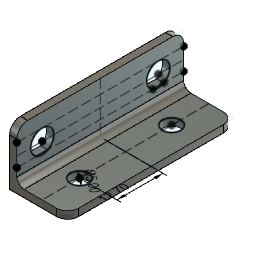
WideBaseAntennaMount (Autodesk Fusion 360 design; units mm, degrees)
Autodesk Fusion 360 part; units mm, degrees
note: some values were not read from the file. Set by a fixed rule: which sketch regions a step uses.
sketch "Sketch1" plane through (0, 0, 0) normal (0, 0, 1) x (1, 0, 0)
  line L0 (0, 0) -> (16, 0)
  line L1 (16, 0) -> (16, 2)
  line L2 (16, 2) -> (2, 2)
  line L3 (2, 2) -> (2, 16)
  line L4 (2, 16) -> (0, 16)
  line L5 (0, 16) -> (0, 0)
  dimension "d1" = 16
  dimension "d2" = 16
  dimension "d3" = 2
  dimension "d4" = 2
  constraint coincident L0.start L5.end
  constraint horizontal L0
  constraint perpendicular L0 L1
  constraint perpendicular L1 L2
  constraint perpendicular L2 L3
  constraint perpendicular L3 L4
  constraint perpendicular L0 L5
  measures "d1" distance of L4.end L0.start
  measures "d2" distance of L0.start L0.end
  measures "d3" distance of L0.end L1.end
  measures "d4" distance of L3.end L4.end
extrude "Extrude1" add sketch "Sketch1" against normal blind 46
sketch "Sketch2" plane through (0, 2, 0) normal (0, 1, 0) x (-1, 0, 0)
  line L0 (-2, 0) -> (-16, 0)
  line L1 (-16, 0) -> (-16, -46)
  line L2 (-16, -46) -> (-2, -46)
  line L3 (-2, -46) -> (-2, 0)
  line L4 (-9, -46) -> (-9, 0) construction
  line L5 (-16, -23) -> (-2, -23) construction
  circle A0 centre (-9, -10.3) radius 2.5
  circle A1 centre (-9, -35.7) radius 2.5
  dimension "d7" = 5
  dimension "d19" = 12.7
  constraint midpoint L2 L4.start
  constraint midpoint L0 L4.end
  constraint midpoint L1 L5.start
  constraint midpoint L3 L5.end
  constraint coincident L4 A0.centre
  constraint symmetric L5 A0 A1
  measures "d7" diameter of A0
  measures "d19" distance of L5 A0.centre
extrude "Extrude2" cut sketch "Sketch2" against normal blind 2 contours A0 | A1
sketch "Sketch3" plane through (2, 0, 0) normal (1, 0, 0) x (0, 0, -1)
  line L0 (0, 16) -> (0, 2)
  line L1 (0, 2) -> (46, 2)
  line L2 (46, 2) -> (46, 16)
  line L3 (46, 16) -> (0, 16)
  line L4 (23, 16) -> (23, 2) construction
  line L5 (0, 9) -> (46, 9) construction
  circle A0 centre (7, 9) radius 3.2
  line L6 (0, 12.2) -> (46, 12.2) construction
  line L7 (0, 6.2) -> (46, 6.2) construction
  line L8 (5.4508, 6.2) -> (8.5492, 6.2)
  circle A1 centre (39, 9) radius 3.2
  line L9 (40.5492, 6.2) -> (37.4508, 6.2)
  dimension "d10" = 6.4
  dimension "d11" = 6
  dimension "d12" = 16
  constraint midpoint L3 L4.start
  constraint midpoint L1 L4.end
  constraint midpoint L0 L5.start
  constraint midpoint L2 L5.end
  constraint coincident L5 A0.centre
  constraint coincident L0 L6.start
  constraint coincident L2 L6.end
  constraint perpendicular L2 L6
  constraint coincident L0 L7.start
  constraint coincident L2 L7.end
  constraint perpendicular L2 L7
  constraint tangent A0 L6
  constraint coincident L7 L8.start
  constraint coincident A0 L8.start
  constraint coincident L7 L8.end
  constraint coincident A0 L8.end
  constraint symmetric L4 A0 A1
  constraint symmetric L4 L8.start L9.start
  constraint symmetric L4 L8.end L9.end
  measures "d10" diameter of A0
  measures "d11" distance of L6 L7
  measures "d12" distance of L4 A0.centre
extrude "Extrude3" cut sketch "Sketch3" against normal blind 2 contours A0 L8 | A1 L9 picked at (6.9734, 8.1997) picked at (38.4662, 7.5792)
fillet "Fillet1" radius 2 1 edges at (2, 2, -23)
fillet "Fillet2" radius 3 4 edges at (1, 16, -46) (1, 16, 0) (16, 1, 0) (16, 1, -46)
equation "d12 = ( 32 / 2 ) * 1 mm"
equation "d19 = ( 25.4 / 2 ) * 1 mm"
